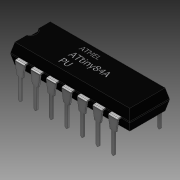
# Autodesk Inventor part: ATtiny84
Saved by Autodesk Inventor 2015 SP1 (Build 190203100, 203)
## iProperties
Created: 2016-08-03
Part Number: ATtiny84
Material: Generisch
Document SubType Name: Modeling
Designer: Gabriel
Density: 1 g/cm^3
Appearance: Eloxiert - schwarz
Author: Gabriel
Autodesk Inventor part; units mm, degrees
ref_plane "YZ Plane" through (0, 0, 0) normal (1, 0, 0) x (0, 1, 0)
sketch "Skizze4" plane through (0, 0, 0) normal (0, 0, 1) x (1, 0, 0)
  line L0 (9.6, -3.2) -> (-9.6, -3.2)
  line L1 (-9.6, -3.2) -> (-9.6, 3.2)
  line L2 (-9.6, 3.2) -> (9.6, 3.2)
  line L3 (9.6, 3.2) -> (9.6, -3.2)
  line L4 (9.6, -3.2) -> (-9.6, 3.2) construction
  line L5 (-9.6, -3.2) -> (9.6, 3.2) construction
  point P0 (0, 0)
  dimension "d15" = 19.2
  dimension "d16" = 6.4
  constraints: 12 end point, 2 midpoint, 2 parallel, 1 horizontal, 1 perpendicular
  measures "d15" distance of L1.end L2.end
  measures "d16" distance of L2.end L0.start
extrude "Extrusion5" add sketch "Skizze4" along normal blind 3.2
chamfer "Fase3" distance 0.35 distance2 1.5 1 edges at (9.6, 0, 3.2) measured on face at (3.2, -1.0667, 3.2)
chamfer "Fase4" distance 0.35 distance2 1.5 1 edges at (9.6, 0, 0) measured on face at (3.2, -1.0667, 0)
chamfer "Fase5" distance 0.35 distance2 1.5 1 edges at (-9.6, 0, 3.2) measured on face at (-3.3167, -1.0667, 3.2)
chamfer "Fase6" distance 0.35 distance2 1.5 1 edges at (-9.6, 0, 0) measured on face at (-3.3167, -1.0667, 0)
chamfer "Fase7" distance 0.35 distance2 1.5 1 edges at (0, 3.2, 0) measured on face at (-3.0833, -1.0667, 0)
chamfer "Fase8" distance 0.35 distance2 1.5 1 edges at (0, 3.2, 3.2) measured on face at (3.0833, 1.0667, 3.2)
chamfer "Fase9" distance 0.35 distance2 1.5 1 edges at (0, -3.2, 3.2) measured on face at (3.0833, 0.8333, 3.2)
chamfer "Fase10" distance 0.35 distance2 1.5 1 edges at (0, -3.2, 0) measured on face at (-3.0833, -1.1833, 0)
sketch "Skizze5" plane through (-9.6, -3.2, 1.7) normal (0, -1, 0) x (1, 0, 0)
  line L0 (19.2, 0) -> (0, 0) projected
  line L1 (0, -0.2) -> (19.2, -0.2) projected
  line L2 (1.35, 0) -> (2.85, 0)
  line L3 (2.85, 0) -> (2.85, -0.2)
  line L4 (2.85, -0.2) -> (1.35, -0.2)
  line L5 (1.35, -0.2) -> (1.35, 0)
  line L6 (3.85, 0) -> (5.35, 0)
  line L7 (5.35, 0) -> (5.35, -0.2)
  line L8 (5.35, -0.2) -> (3.85, -0.2)
  line L9 (3.85, -0.2) -> (3.85, 0)
  line L10 (6.35, 0) -> (7.85, 0)
  line L11 (7.85, 0) -> (7.85, -0.2)
  line L12 (7.85, -0.2) -> (6.35, -0.2)
  line L13 (6.35, -0.2) -> (6.35, 0)
  line L14 (8.85, 0) -> (10.35, 0)
  line L15 (10.35, 0) -> (10.35, -0.2)
  line L16 (10.35, -0.2) -> (8.85, -0.2)
  line L17 (8.85, -0.2) -> (8.85, 0)
  line L18 (11.35, 0) -> (12.85, 0)
  line L19 (12.85, 0) -> (12.85, -0.2)
  line L20 (12.85, -0.2) -> (11.35, -0.2)
  line L21 (11.35, -0.2) -> (11.35, 0)
  line L22 (13.85, 0) -> (15.35, 0)
  line L23 (15.35, 0) -> (15.35, -0.2)
  line L24 (15.35, -0.2) -> (13.85, -0.2)
  line L25 (13.85, -0.2) -> (13.85, 0)
  line L26 (16.35, 0) -> (17.85, 0)
  line L27 (17.85, 0) -> (17.85, -0.2)
  line L28 (17.85, -0.2) -> (16.35, -0.2)
  line L29 (16.35, -0.2) -> (16.35, 0)
  line L30 (9.6, -4.1914) -> (9.6, 2.6065) construction
  line L31 (18.85, 1.5) -> (0.35, 1.5) construction
  point P0 (9.6, -1.7)
  point P1 (9.6, 1.5)
  dimension "d43" = 1.5
  dimension "d44" = 1.5
  dimension "d45" = 1.5
  dimension "d46" = 1.5
  dimension "d47" = 1.5
  dimension "d48" = 1.5
  dimension "d49" = 1.5
  dimension "d51" = 4
  dimension "d52" = 4
  dimension "d53" = 4
  dimension "d54" = 4
  dimension "d55" = 4
  dimension "d56" = 4
  constraints: 58 end point, 14 parallel, 7 horizontal, 7 perpendicular, 1 midpoint, 1 point on line, 1 vertical, 17 other
  measures "d43" distance between parallel lines of L5 L3
  measures "d44" distance between parallel lines of L7 L9
  measures "d45" distance between parallel lines of L11 L13
  measures "d46" distance between parallel lines of L15 L17
  measures "d47" distance between parallel lines of L19 L21
  measures "d48" distance from line of L23 L22.start
  measures "d49" distance between parallel lines of L27 L29
  measures "d51" distance between parallel lines of L5 L7
  measures "d52" distance between parallel lines of L11 L9
  measures "d53" distance between parallel lines of L15 L13
  measures "d54" distance between parallel lines of L19 L17
  measures "d55" distance between parallel lines of L23 L21
  measures "d56" distance between parallel lines of L27 L25
ref_plane "Arbeitsebene2" through (-8.25, -3.2, 1.7) normal (-1, 0, 0) x (0, 0, 1)
sketch "Skizze6" plane through (-8.25, -3.2, 1.7) normal (-1, 0, 0) x (0, 0, 1)
  line L0 (0, 0) -> (0, -0.5) construction
  line L1 (-0.2, 0) -> (-0.2, -0.5)
  arc A0 (-0.3, -0.8) -> (0, -0.5) centre (-0.3, -0.5) ccw construction
  arc A1 (-0.3, -0.6) -> (-0.2, -0.5) centre (-0.3, -0.5) ccw
  line L2 (-0.2, 0) -> (0, 0) construction
  point P0 (-1.7, 3.2)
  dimension "d57" = 0.8
  dimension "d58" = 0.1
  constraints: 4 end point, 4 point on circle, 2 centre point, 2 coincident, 2 tangent, 2 vertical, 2 vertical alignment
  measures "d57" vertical distance of A0.start L0.start
  measures "d58" distance of A1.start A0.centre
ref_plane "Arbeitsebene4" through (-8.25, -3.8, 1.4) normal (0, -1, 0) x (1, 0, 0)
sketch "Skizze8" plane through (-8.25, -3.8, 1.4) normal (0, -1, 0) x (1, 0, 0)
  line L0 (0.75, -0.391) -> (0.75, 0.6304) construction
  line L1 (0, 0.3) -> (1.5, 0.3) construction
  line L2 (0, 0) -> (0.2374, -1.6145)
  line L3 (1.2626, -1.6145) -> (1.5, 0)
  line L4 (0.5, -1.8) -> (0.5, -5.2)
  line L5 (1, -5.2) -> (1, -1.8)
  line L6 (0.3364, -1.7) -> (0.4, -1.7)
  line L7 (1.1, -1.7) -> (1.1636, -1.7)
  arc A0 (0.2374, -1.6145) -> (0.3364, -1.7) centre (0.3364, -1.6) ccw
  arc A1 (0.5, -1.8) -> (0.4, -1.7) centre (0.4, -1.8) ccw
  arc A2 (1.1, -1.7) -> (1, -1.8) centre (1.1, -1.8) ccw
  arc A3 (1.1636, -1.7) -> (1.2626, -1.6145) centre (1.1636, -1.6) ccw
  line L8 (0.5, -5.2) -> (1, -5.2)
  line L9 (0, 0) -> (0, 0.3)
  line L10 (1.5, 0.3) -> (0, 0.3)
  line L11 (1.5, 0.3) -> (1.5, 0)
  point P0 (8.25, -1.4)
  point P1 (0.25, -1.7)
  point P2 (1.25, -1.7)
  point P3 (0.75, 0.3)
  dimension "d61" = 1
  dimension "d62" = 2
  dimension "d63" = 0.5
  dimension "d65" = 0.1
  dimension "d66" = 5.5
  constraints: 22 end point, 8 point on circle, 8 tangent, 6 point on line, 4 centre point, 3 collinear, 3 equal radius, 3 vertical, 2 horizontal, 2 perpendicular, 1 horizontal alignment, 1 midpoint, 1 symmetric about line
  measures "d61" distance of point (0.25, -1.7) point (1.25, -1.7)
  measures "d62" distance from line of L1 point (0.25, -1.7)
  measures "d63" distance of L4.end L5.start
  measures "d65" radius of A0
  measures "d66" distance from line of L1 L4.end
extrude "Extrusion6" add sketch "Skizze8" against normal blind 0.2
extrude "Extrusion7" add sketch "Skizze5" along normal blind 0.5 contours L3 L1 L5 L0
fillet "Rundung1" radius 0.2 1 edges at (-7.5, -3.8, 1.7)
fillet "Rundung2" radius 0.1 1 edges at (-7.5, -3.6, 1.5)
chamfer "Fase11" distance 0.2 angle 45 2 edges at (-7.75, -3.7, -3.8) (-7.25, -3.7, -3.8)
pattern_linear "Rechteckige Anordnung1" count 7 spacing 2.5 along (1, 0, 0) of "Extrusion6", "Extrusion7", "Rundung1", "Rundung2", "Fase11"
mirror "Spiegeln1" about plane through (0, 0, 0) normal (0, 1, 0) of "Extrusion6", "Extrusion7", "Rundung1", "Rundung2", "Fase11", "Rechteckige Anordnung1"
sketch "Skizze10" plane through (0, 0, 3.2) normal (0, 0, 1) x (1, 0, 0)
  circle A0 centre (-9.6, 0) radius 1
  line L0 (-9.6, 3.2) -> (-9.6, -3.2) projected
  point P0 (0, 0)
  dimension "d80" = 2
  constraints: 1 centre point, 1 midpoint
  measures "d80" diameter of A0
extrude "Extrusion8" cut sketch "Skizze10" against normal blind 0.5
sketch "Skizze11" plane through (0, 0, 3.2) normal (0, 0, 1) x (1, 0, 0)
  line L0 (-3.161, 2.0624) -> (4.8997, 2.0624) construction
  line L1 (4.8997, 2.0624) -> (4.8997, 1.314) construction
  line L2 (4.8997, 1.314) -> (-3.161, 1.314) construction
  line L3 (-3.161, 1.314) -> (-3.161, 2.0624) construction
  line L4 (-3.161, 0.5897) -> (4.8997, 0.5897) construction
  line L5 (4.8997, 0.5897) -> (4.8997, -3.8631) construction
  line L6 (4.8997, -3.8631) -> (-3.161, -3.8631) construction
  line L7 (-3.161, -3.8631) -> (-3.161, 0.5897) construction
  line L8 (-3.1658, 1.3124) -> (-2.913, 2.0624)
  line L9 (-2.913, 2.0624) -> (-2.7902, 2.0624)
  line L10 (-2.7902, 2.0624) -> (-2.5374, 1.3124)
  line L11 (-2.5374, 1.3124) -> (-2.6425, 1.3124)
  line L12 (-2.6425, 1.3124) -> (-2.7106, 1.5221)
  line L13 (-2.7106, 1.5221) -> (-2.9969, 1.5221)
  line L14 (-2.9969, 1.5221) -> (-3.0649, 1.3124)
  line L15 (-3.0649, 1.3124) -> (-3.1658, 1.3124)
  line L16 (-2.7379, 1.6072) -> (-2.854, 1.9603)
  line L17 (-2.854, 1.9603) -> (-2.9695, 1.6072)
  line L18 (-2.9695, 1.6072) -> (-2.7379, 1.6072)
  line L19 (-2.2912, 1.3124) -> (-2.2912, 1.9737)
  line L20 (-2.2912, 1.9737) -> (-2.5428, 1.9737)
  line L21 (-2.5428, 1.9737) -> (-2.5428, 2.0624)
  line L22 (-2.5428, 2.0624) -> (-1.9399, 2.0624)
  line L23 (-1.9399, 2.0624) -> (-1.9399, 1.9737)
  line L24 (-1.9399, 1.9737) -> (-2.1916, 1.9737)
  line L25 (-2.1916, 1.9737) -> (-2.1916, 1.3124)
  line L26 (-2.1916, 1.3124) -> (-2.2912, 1.3124)
  line L27 (-1.2209, 1.3124) -> (-1.3206, 1.3124)
  line L28 (-1.3206, 1.3124) -> (-1.3206, 1.9585)
  line L29 (-1.3206, 1.9585) -> (-1.5163, 1.5191)
  line L30 (-1.5163, 1.5191) -> (-1.5771, 1.5191)
  line L31 (-1.5771, 1.5191) -> (-1.771, 1.9585)
  line L32 (-1.771, 1.9585) -> (-1.771, 1.3124)
  line L33 (-1.771, 1.3124) -> (-1.864, 1.3124)
  line L34 (-1.864, 1.3124) -> (-1.864, 2.0624)
  line L35 (-1.864, 2.0624) -> (-1.7278, 2.0624)
  line L36 (-1.7278, 2.0624) -> (-1.5406, 1.6449)
  line L37 (-1.5406, 1.6449) -> (-1.3595, 2.0624)
  line L38 (-1.3595, 2.0624) -> (-1.2209, 2.0624)
  line L39 (-1.2209, 2.0624) -> (-1.2209, 1.3124)
  line L40 (-1.069, 1.3124) -> (-1.069, 2.0624)
  line L41 (-1.069, 2.0624) -> (-0.5998, 2.0624)
  line L42 (-0.5998, 2.0624) -> (-0.5998, 1.9737)
  line L43 (-0.5998, 1.9737) -> (-0.9693, 1.9737)
  line L44 (-0.9693, 1.9737) -> (-0.9693, 1.7683)
  line L45 (-0.9693, 1.7683) -> (-0.6247, 1.7683)
  line L46 (-0.6247, 1.7683) -> (-0.6247, 1.6795)
  line L47 (-0.6247, 1.6795) -> (-0.9693, 1.6795)
  line L48 (-0.9693, 1.6795) -> (-0.9693, 1.4012)
  line L49 (-0.9693, 1.4012) -> (-0.5998, 1.4012)
  line L50 (-0.5998, 1.4012) -> (-0.5998, 1.3124)
  line L51 (-0.5998, 1.3124) -> (-1.069, 1.3124)
  line L52 (-0.0558, 1.3124) -> (-0.4904, 1.3124)
  line L53 (-0.4904, 1.3124) -> (-0.4904, 2.0624)
  line L54 (-0.4904, 2.0624) -> (-0.3907, 2.0624)
  line L55 (-0.3907, 2.0624) -> (-0.3907, 1.4012)
  line L56 (-0.3907, 1.4012) -> (-0.0558, 1.4012)
  line L57 (-0.0558, 1.4012) -> (-0.0558, 1.3124)
  line L58 (-3.1674, -0.433) -> (-2.8303, 0.567)
  line L59 (-2.8303, 0.567) -> (-2.6666, 0.567)
  line L60 (-2.6666, 0.567) -> (-2.3295, -0.433)
  line L61 (-2.3295, -0.433) -> (-2.4697, -0.433)
  line L62 (-2.4697, -0.433) -> (-2.5605, -0.1534)
  line L63 (-2.5605, -0.1534) -> (-2.9422, -0.1534)
  line L64 (-2.9422, -0.1534) -> (-3.0329, -0.433)
  line L65 (-3.0329, -0.433) -> (-3.1674, -0.433)
  line L66 (-2.5969, -0.0399) -> (-2.7517, 0.4309)
  line L67 (-2.7517, 0.4309) -> (-2.9057, -0.0399)
  line L68 (-2.9057, -0.0399) -> (-2.5969, -0.0399)
  line L69 (-2.0013, -0.433) -> (-2.0013, 0.4487)
  line L70 (-2.0013, 0.4487) -> (-2.3368, 0.4487)
  line L71 (-2.3368, 0.4487) -> (-2.3368, 0.567)
  line L72 (-2.3368, 0.567) -> (-1.5329, 0.567)
  line L73 (-1.5329, 0.567) -> (-1.5329, 0.4487)
  line L74 (-1.5329, 0.4487) -> (-1.8684, 0.4487)
  line L75 (-1.8684, 0.4487) -> (-1.8684, -0.433)
  line L76 (-1.8684, -0.433) -> (-2.0013, -0.433)
  spline S0 degree 2 poles (-1.2144, -0.4476) (-1.3174, -0.4476) (-1.4332, -0.3301) (-1.4332, -0.2028) knots 0 0 0 1 2 2 2
  line L77 (-1.4332, -0.2028) -> (-1.4332, 0.2129)
  line L78 (-1.4332, 0.2129) -> (-1.5183, 0.2129)
  line L79 (-1.5183, 0.2129) -> (-1.5183, 0.3174)
  line L80 (-1.5183, 0.3174) -> (-1.4332, 0.3174)
  line L81 (-1.4332, 0.3174) -> (-1.4332, 0.533)
  line L82 (-1.4332, 0.533) -> (-1.3068, 0.533)
  line L83 (-1.3068, 0.533) -> (-1.3068, 0.3174)
  line L84 (-1.3068, 0.3174) -> (-1.0742, 0.3174)
  line L85 (-1.0742, 0.3174) -> (-1.0742, 0.2129)
  line L86 (-1.0742, 0.2129) -> (-1.3068, 0.2129)
  line L87 (-1.3068, 0.2129) -> (-1.3068, -0.1445)
  spline S1 degree 2 poles (-1.3068, -0.1445) (-1.3068, -0.2012) (-1.3028, -0.2636) (-1.289, -0.2903) knots 0 0 0 1 2 2 2
  spline S2 degree 2 poles (-1.289, -0.2903) (-1.2777, -0.3138) (-1.2266, -0.3373) (-1.1828, -0.3373) knots 0 0 0 1 2 2 2
  spline S3 degree 2 poles (-1.1828, -0.3373) (-1.152, -0.3373) (-1.0945, -0.3187) (-1.0815, -0.313) knots 0 0 0 1 2 2 2
  line L88 (-1.0815, -0.313) -> (-1.0742, -0.313)
  line L89 (-1.0742, -0.313) -> (-1.0742, -0.4265)
  spline S4 degree 2 poles (-1.0742, -0.4265) (-1.1099, -0.4362) (-1.1828, -0.4476) (-1.2144, -0.4476) knots 0 0 0 1 2 2 2
  line L90 (-0.8522, -0.433) -> (-0.9786, -0.433)
  line L91 (-0.9786, -0.433) -> (-0.9786, 0.3174)
  line L92 (-0.9786, 0.3174) -> (-0.8522, 0.3174)
  line L93 (-0.8522, 0.3174) -> (-0.8522, -0.433)
  line L94 (-0.8433, 0.4422) -> (-0.9867, 0.4422)
  line L95 (-0.9867, 0.4422) -> (-0.9867, 0.5735)
  line L96 (-0.9867, 0.5735) -> (-0.8433, 0.5735)
  line L97 (-0.8433, 0.5735) -> (-0.8433, 0.4422)
  line L98 (-0.0775, -0.433) -> (-0.2039, -0.433)
  line L99 (-0.2039, -0.433) -> (-0.2039, -0.0051)
  spline S5 degree 2 poles (-0.2039, -0.0051) (-0.2039, 0.0468) (-0.2136, 0.1359) (-0.2282, 0.1627) knots 0 0 0 1 2 2 2
  spline S6 degree 2 poles (-0.2282, 0.1627) (-0.2436, 0.191) (-0.2987, 0.2186) (-0.3457, 0.2186) knots 0 0 0 1 2 2 2
  spline S7 degree 2 poles (-0.3457, 0.2186) (-0.3927, 0.2186) (-0.4924, 0.1683) (-0.5402, 0.1278) knots 0 0 0 1 2 2 2
  line L100 (-0.5402, 0.1278) -> (-0.5402, -0.433)
  line L101 (-0.5402, -0.433) -> (-0.6666, -0.433)
  line L102 (-0.6666, -0.433) -> (-0.6666, 0.3174)
  line L103 (-0.6666, 0.3174) -> (-0.5402, 0.3174)
  line L104 (-0.5402, 0.3174) -> (-0.5402, 0.234)
  spline S8 degree 2 poles (-0.5402, 0.234) (-0.4835, 0.285) (-0.3741, 0.3385) (-0.3125, 0.3385) knots 0 0 0 1 2 2 2
  spline S9 degree 2 poles (-0.3125, 0.3385) (-0.2023, 0.3385) (-0.0775, 0.1926) (-0.0775, 0.0541) knots 0 0 0 1 2 2 2
  line L105 (-0.0775, 0.0541) -> (-0.0775, -0.433)
  line L106 (0.6891, 0.3174) -> (0.2856, -0.7093)
  line L107 (0.2856, -0.7093) -> (0.1502, -0.7093)
  line L108 (0.1502, -0.7093) -> (0.2847, -0.3965)
  line L109 (0.2847, -0.3965) -> (0.0125, 0.3174)
  line L110 (0.0125, 0.3174) -> (0.1486, 0.3174)
  line L111 (0.1486, 0.3174) -> (0.3536, -0.2385)
  line L112 (0.3536, -0.2385) -> (0.5578, 0.3174)
  line L113 (0.5578, 0.3174) -> (0.6891, 0.3174)
  spline S10 degree 2 poles (1.0684, -0.4557) (0.9938, -0.4557) (0.8715, -0.4111) (0.8285, -0.3698) knots 0 0 0 1 2 2 2
  spline S11 degree 2 poles (0.8285, -0.3698) (0.7864, -0.3292) (0.7426, -0.219) (0.7426, -0.1566) knots 0 0 0 1 2 2 2
  spline S12 degree 2 poles (0.7426, -0.1566) (0.7426, -0.0756) (0.8293, 0.0605) (0.912, 0.1011) knots 0 0 0 1 2 2 2
  line L114 (0.912, 0.1011) -> (0.912, 0.1051)
  spline S13 degree 2 poles (0.912, 0.1051) (0.8382, 0.1481) (0.7669, 0.2502) (0.7669, 0.3263) knots 0 0 0 1 2 2 2
  spline S14 degree 2 poles (0.7669, 0.3263) (0.7669, 0.439) (0.9371, 0.5897) (1.0684, 0.5897) knots 0 0 0 1 2 2 2
  spline S15 degree 2 poles (1.0684, 0.5897) (1.2045, 0.5897) (1.369, 0.4471) (1.369, 0.3353) knots 0 0 0 1 2 2 2
  spline S16 degree 2 poles (1.369, 0.3353) (1.369, 0.268) (1.2904, 0.1367) (1.2167, 0.0994) knots 0 0 0 1 2 2 2
  line L115 (1.2167, 0.0994) -> (1.2167, 0.0954)
  spline S17 degree 2 poles (1.2167, 0.0954) (1.3042, 0.0549) (1.3941, -0.0618) (1.3941, -0.1542) knots 0 0 0 1 2 2 2
  spline S18 degree 2 poles (1.3941, -0.1542) (1.3941, -0.2822) (1.2078, -0.4557) (1.0684, -0.4557) knots 0 0 0 1 2 2 2
  spline S19 degree 2 poles (1.2564, -0.1672) (1.2564, -0.1056) (1.2078, -0.0326) (1.1389, 0.0046) knots 0 0 0 1 2 2 2
  spline S20 degree 2 poles (1.1389, 0.0046) (1.1162, 0.0176) (1.04, 0.0476) (0.9922, 0.067) knots 0 0 0 1 2 2 2
  spline S21 degree 2 poles (0.9922, 0.067) (0.9371, 0.0306) (0.8779, -0.078) (0.8779, -0.1469) knots 0 0 0 1 2 2 2
  spline S22 degree 2 poles (0.8779, -0.1469) (0.8779, -0.2377) (0.9873, -0.356) (1.07, -0.356) knots 0 0 0 1 2 2 2
  spline S23 degree 2 poles (1.07, -0.356) (1.1543, -0.356) (1.2564, -0.2547) (1.2564, -0.1672) knots 0 0 0 1 2 2 2
  spline S24 degree 2 poles (1.2377, 0.3336) (1.2377, 0.4009) (1.1478, 0.4909) (1.0676, 0.4909) knots 0 0 0 1 2 2 2
  spline S25 degree 2 poles (1.0676, 0.4909) (0.9946, 0.4909) (0.9014, 0.4106) (0.9014, 0.3417) knots 0 0 0 1 2 2 2
  spline S26 degree 2 poles (0.9014, 0.3417) (0.9014, 0.2923) (0.9493, 0.2234) (0.9971, 0.1959) knots 0 0 0 1 2 2 2
  spline S27 degree 2 poles (0.9971, 0.1959) (1.0173, 0.1845) (1.1032, 0.1448) (1.1381, 0.1335) knots 0 0 0 1 2 2 2
  spline S28 degree 2 poles (1.1381, 0.1335) (1.1964, 0.178) (1.2377, 0.2729) (1.2377, 0.3336) knots 0 0 0 1 2 2 2
  line L116 (2.1599, -0.0894) -> (2.0408, -0.0894)
  line L117 (2.0408, -0.0894) -> (2.0408, -0.433)
  line L118 (2.0408, -0.433) -> (1.912, -0.433)
  line L119 (1.912, -0.433) -> (1.912, -0.0894)
  line L120 (1.912, -0.0894) -> (1.4703, -0.0894)
  line L121 (1.4703, -0.0894) -> (1.4703, 0.0516)
  line L122 (1.4703, 0.0516) -> (1.9176, 0.567)
  line L123 (1.9176, 0.567) -> (2.0408, 0.567)
  line L124 (2.0408, 0.567) -> (2.0408, 0.0184)
  line L125 (2.0408, 0.0184) -> (2.1599, 0.0184)
  line L126 (2.1599, 0.0184) -> (2.1599, -0.0894)
  line L127 (1.912, 0.0184) -> (1.912, 0.409)
  line L128 (1.912, 0.409) -> (1.5757, 0.0184)
  line L129 (1.5757, 0.0184) -> (1.912, 0.0184)
  line L130 (2.1875, -0.433) -> (2.5246, 0.567)
  line L131 (2.5246, 0.567) -> (2.6883, 0.567)
  line L132 (2.6883, 0.567) -> (3.0254, -0.433)
  line L133 (3.0254, -0.433) -> (2.8852, -0.433)
  line L134 (2.8852, -0.433) -> (2.7945, -0.1534)
  line L135 (2.7945, -0.1534) -> (2.4128, -0.1534)
  line L136 (2.4128, -0.1534) -> (2.322, -0.433)
  line L137 (2.322, -0.433) -> (2.1875, -0.433)
  line L138 (2.758, -0.0399) -> (2.6032, 0.4309)
  line L139 (2.6032, 0.4309) -> (2.4493, -0.0399)
  line L140 (2.4493, -0.0399) -> (2.758, -0.0399)
  spline S29 degree 2 poles (-2.4276, -1.3809) (-2.4276, -1.4457) (-2.4738, -1.5624) (-2.5151, -1.6029) knots 0 0 0 1 2 2 2
  spline S30 degree 2 poles (-2.5151, -1.6029) (-2.567, -1.654) (-2.7072, -1.7067) (-2.8141, -1.7067) knots 0 0 0 1 2 2 2
  line L141 (-2.8141, -1.7067) -> (-2.9268, -1.7067)
  line L142 (-2.9268, -1.7067) -> (-2.9268, -2.0794)
  line L143 (-2.9268, -2.0794) -> (-3.0597, -2.0794)
  line L144 (-3.0597, -2.0794) -> (-3.0597, -1.0794)
  line L145 (-3.0597, -1.0794) -> (-2.8084, -1.0794)
  spline S31 degree 2 poles (-2.8084, -1.0794) (-2.7193, -1.0794) (-2.5945, -1.1086) (-2.5467, -1.1418) knots 0 0 0 1 2 2 2
  spline S32 degree 2 poles (-2.5467, -1.1418) (-2.4908, -1.1799) (-2.4276, -1.2974) (-2.4276, -1.3809) knots 0 0 0 1 2 2 2
  spline S33 degree 2 poles (-2.5661, -1.385) (-2.5661, -1.3331) (-2.6018, -1.2569) (-2.6383, -1.2326) knots 0 0 0 1 2 2 2
  spline S34 degree 2 poles (-2.6383, -1.2326) (-2.6699, -1.2115) (-2.7542, -1.1945) (-2.8166, -1.1945) knots 0 0 0 1 2 2 2
  line L146 (-2.8166, -1.1945) -> (-2.9268, -1.1945)
  line L147 (-2.9268, -1.1945) -> (-2.9268, -1.5932)
  line L148 (-2.9268, -1.5932) -> (-2.836, -1.5932)
  spline S35 degree 2 poles (-2.836, -1.5932) (-2.755, -1.5932) (-2.6553, -1.5673) (-2.6229, -1.5333) knots 0 0 0 1 2 2 2
  spline S36 degree 2 poles (-2.6229, -1.5333) (-2.5929, -1.5033) (-2.5661, -1.4328) (-2.5661, -1.385) knots 0 0 0 1 2 2 2
  spline S37 degree 2 poles (-1.9519, -2.1005) (-2.0402, -2.1005) (-2.1715, -2.0543) (-2.2177, -2.0081) knots 0 0 0 1 2 2 2
  spline S38 degree 2 poles (-2.2177, -2.0081) (-2.2704, -1.9563) (-2.3133, -1.8104) (-2.3133, -1.7034) knots 0 0 0 1 2 2 2
  line L149 (-2.3133, -1.7034) -> (-2.3133, -1.0794)
  line L150 (-2.3133, -1.0794) -> (-2.1804, -1.0794)
  line L151 (-2.1804, -1.0794) -> (-2.1804, -1.7034)
  spline S39 degree 2 poles (-2.1804, -1.7034) (-2.1804, -1.7731) (-2.1626, -1.8671) (-2.1375, -1.9052) knots 0 0 0 1 2 2 2
  spline S40 degree 2 poles (-2.1375, -1.9052) (-2.1107, -1.9457) (-2.0183, -1.9871) (-1.9519, -1.9871) knots 0 0 0 1 2 2 2
  spline S41 degree 2 poles (-1.9519, -1.9871) (-1.8895, -1.9871) (-1.7922, -1.9457) (-1.7655, -1.9052) knots 0 0 0 1 2 2 2
  spline S42 degree 2 poles (-1.7655, -1.9052) (-1.7404, -1.8671) (-1.7225, -1.7739) (-1.7225, -1.7067) knots 0 0 0 1 2 2 2
  line L152 (-1.7225, -1.7067) -> (-1.7225, -1.0794)
  line L153 (-1.7225, -1.0794) -> (-1.5896, -1.0794)
  line L154 (-1.5896, -1.0794) -> (-1.5896, -1.7034)
  spline S43 degree 2 poles (-1.5896, -1.7034) (-1.5896, -1.808) (-1.6318, -1.9571) (-1.6853, -2.0081) knots 0 0 0 1 2 2 2
  spline S44 degree 2 poles (-1.6853, -2.0081) (-1.7331, -2.0551) (-1.8595, -2.1005) (-1.9519, -2.1005) knots 0 0 0 1 2 2 2
  point P0 (0, 0)
  constraints: 1 collinear, 4 other
extrude "Extrusion9" cut sketch "Skizze11" against normal blind 0.01
